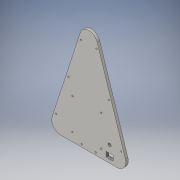
# Autodesk Inventor part: Nathan_LED_Speaker_Back
Saved by Autodesk Inventor 2016 (Build 200138000, 138)
## iProperties
Created: 2018-09-27
Part Number: Nathan_LED_Speaker_Back
Material: Generic
Document SubType Name: Modeling
Designer: Student
Density: 1 g/cm^3
Appearance: Default
Author: Student
Autodesk Inventor part; units mm, degrees
ref_plane "YZ Plane" through (0, 0, 0) normal (1, 0, 0) x (0, 1, 0)
ref_plane "XZ Plane" through (0, 0, 0) normal (0, 1, 0) x (-1, 0, 0)
ref_plane "XY Plane" through (0, 0, 0) normal (0, 0, 1) x (1, 0, 0)
sketch "Sketch1" plane through (0, 0, 0) normal (0, 0, 1) x (1, 0, 0)
  arc A0 (-2.4007, 17.5975) -> (12.7, -3.175) centre (12.7, 12.7) ccw
  arc A1 (114.3, -3.175) -> (129.4007, 17.5975) centre (114.3, 12.7) ccw
  line L0 (114.3, -3.175) -> (12.7, -3.175)
  line L1 (48.3993, 174.2307) -> (-2.4007, 17.5975)
  line L2 (129.4007, 17.5975) -> (78.6007, 174.2307)
  arc A2 (78.6007, 174.2307) -> (48.3993, 174.2307) centre (63.5, 169.3332) ccw
  arc A3 (75.5805, 173.2512) -> (51.4195, 173.2512) centre (63.5, 169.3332) ccw
  arc A4 (0.6195, 16.618) -> (12.7, 0) centre (12.7, 12.7) ccw
  arc A5 (114.3, 0) -> (126.3805, 16.618) centre (114.3, 12.7) ccw
  line L3 (12.7, 0) -> (114.3, 0)
  line L4 (0.6195, 16.618) -> (51.4195, 173.2512)
  line L5 (75.5805, 173.2512) -> (126.3805, 16.618)
  line L6 (0.6195, 16.618) -> (3.7539, 26.2824)
  line L7 (3.7539, 26.2824) -> (4.9619, 25.8906)
  circle A6 centre (4.9619, 25.8906) radius 1.27
  line L8 (51.4195, 173.2512) -> (48.2851, 163.5868)
  line L9 (48.2851, 163.5868) -> (49.4931, 163.195)
  circle A7 centre (49.4931, 163.195) radius 1.27
  circle A8 centre (27.2275, 94.5428) radius 1.27
  line L10 (75.5805, 173.2512) -> (78.7149, 163.5868)
  line L11 (78.7149, 163.5868) -> (77.5069, 163.195)
  circle A9 centre (77.5069, 163.195) radius 1.27
  line L12 (126.3805, 16.618) -> (123.2461, 26.2824)
  line L13 (123.2461, 26.2824) -> (122.0381, 25.8906)
  circle A10 centre (122.0381, 25.8906) radius 1.27
  circle A11 centre (99.7725, 94.5428) radius 1.27
  line L14 (63.5, 0) -> (63.5, 1.27) construction
  line L15 (63.5, 1.27) -> (76.2, 1.27) construction
  line L16 (63.5, 1.27) -> (50.8, 1.27) construction
  circle A12 centre (50.8, 1.27) radius 1.27
  circle A13 centre (76.2, 1.27) radius 1.27
  point P0 (0, 0)
  point P1 (0, 0)
  dimension "d50" = 2.54
  dimension "d53" = 2.54
  dimension "d39" = 31.75
  dimension "d40" = 31.75
  dimension "d41" = 25.4
  dimension "d42" = 25.4
  dimension "d43" = 25.4
  dimension "d44" = 10.16
  dimension "d45" = 10.16
  dimension "d46" = 1.27
  dimension "d47" = 1.27
  dimension "d48" = 10.16
  dimension "d49" = 10.16
  dimension "d51" = 2.54
  dimension "d52" = 2.54
  dimension "d91" = 12.7
  dimension "d92" = 12.7
  constraints: 34 end point, 12 point on circle, 10 centre point, 9 coincident, 6 tangent, 4 point on line, 2 perpendicular, 1 horizontal, 1 midpoint, 12 other
  measures "d39" diameter of A0
  measures "d40" diameter of A1
  measures "d41" diameter of A3
  measures "d42" diameter of A4
  measures "d43" diameter of A5
  measures "d44" distance of L4.start L7.start
  measures "d45" distance of L4.end L9.start
  measures "d46" distance of L9.start L9.end
  measures "d47" distance of L11.start L11.end
  measures "d48" distance of L5.end L12.end
  measures "d49" distance of L11.start L5.start
  measures "d51" diameter of A8
  measures "d52" diameter of A11
  measures "d91" distance of L14.end L15.end
  measures "d92" distance of L14.end L16.end
ref_plane "Work Plane1" through (0, 0, 4.572) normal (0, 0, 1) x (1, 0, 0)
sketch "Sketch2" plane through (0, 0, 4.572) normal (0, 0, 1) x (1, 0, 0)
  line L0 (12.7, -3.175) -> (114.3, -3.175) projected
  line L1 (34.1719, 12.065) -> (34.1719, 67.945) construction
  line L2 (34.1719, 67.945) -> (86.2419, 67.945) construction
  line L3 (86.2419, 67.945) -> (86.2419, 12.065) construction
  line L4 (86.2419, 12.065) -> (34.1719, 12.065) construction
  line L5 (34.1719, 12.065) -> (86.2419, 67.945) construction
  line L6 (34.1719, 67.945) -> (86.2419, 12.065) construction
  circle A0 centre (34.1719, 67.945) radius 1.27
  circle A1 centre (34.1719, 12.065) radius 1.27
  circle A2 centre (86.2419, 12.065) radius 1.27
  circle A3 centre (86.2419, 67.945) radius 1.27
  circle A4 centre (4.9619, 25.8906) radius 1.27 projected
  arc A5 (78.6007, 174.2307) -> (48.3993, 174.2307) centre (63.5, 169.3332) ccw projected
  point P0 (0, 0)
  point P1 (60.2069, 40.005)
  dimension "d71" = 55.88
  dimension "d73" = 52.07
  dimension "d74" = 2.54
  dimension "d75" = 2.54
  dimension "d76" = 2.54
  dimension "d77" = 2.54
  dimension "d80" = 52.07
  dimension "d81" = 15.24
  dimension "d82" = 29.21
  constraints: 12 end point, 4 centre point, 4 coincident, 2 midpoint, 2 parallel, 1 perpendicular
  measures "d71" distance of L1.start L1.end
  measures "d73" distance of L1.end L2.end
  measures "d74" diameter of A0
  measures "d75" diameter of A1
  measures "d76" diameter of A2
  measures "d77" diameter of A3
  measures "d80" distance of A2.centre A1.centre
  measures "d81" distance between parallel lines of L4 L0
  measures "d82" distance from line of A4.centre L1
extrude "Extrusion8" add sketch "Sketch1" along normal blind 4.572 contours L1 A2 L2 A1 L0 A0 | L5 A5 L3 A4 L4 A3
sketch "Sketch3" plane through (0, 0, 4.572) normal (0, 0, 1) x (1, 0, 0)
  circle A0 centre (76.2, 1.27) radius 1.27 projected
  line L0 (76.2, 1.27) -> (117.4054, 1.27)
  line L1 (117.4054, 1.27) -> (117.4054, 3.556)
  line L2 (117.4054, 3.556) -> (76.2, 3.556)
  line L3 (76.2, 3.556) -> (76.2, 1.27)
  line L4 (94.8275, 3.556) -> (107.5275, 3.556)
  line L5 (107.5275, 3.556) -> (107.5275, 12.446)
  line L6 (107.5275, 12.446) -> (94.8275, 12.446)
  line L7 (94.8275, 12.446) -> (94.8275, 3.556)
  circle A1 centre (101.1775, 25.5037) radius 2.794
  line L8 (12.7, -3.175) -> (114.3, -3.175) projected
  line L9 (63.5, -3.175) -> (63.5, 31.7936) construction
  line L10 (101.1775, 8.001) -> (63.5, 8.001) construction
  point P0 (0, 0)
  dimension "d97" = 2.286
  dimension "d98" = 12.7
  dimension "d99" = 8.89
  dimension "d106" = 5.588
  dimension "d109" = 37.6775
  constraints: 20 end point, 4 parallel, 3 perpendicular, 2 horizontal, 2 point on line, 1 centre point, 1 midpoint, 1 vertical
  measures "d97" distance of L1.end L0.end
  measures "d98" distance of L6.end L5.end
  measures "d99" distance of L5.end L4.end
  measures "d106" diameter of A1
  measures "d109" distance of L10.start L10.end
extrude "Extrusion10" cut sketch "Sketch3" against normal blind 25.4 contours L7 L6 L5 L2 | A1
fillet "Fillet1" radius 0.635 1 edges at (94.8275, 12.446, 2.286)
fillet "Fillet2" radius 0.635 1 edges at (107.5275, 12.446, 2.286)
fillet "Fillet3" radius 0.635 1 edges at (94.8275, 3.556, 2.286)
fillet "Fillet4" radius 0.635 1 edges at (107.5275, 3.556, 2.286)
extrude "Extrusion11" cut sketch "Sketch2" against normal blind 25.4 contours A0 | A1 | A2 | A3
body "Solid5"
